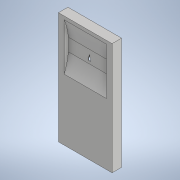
# Autodesk Inventor part: Mosquito Holder v12 RU - Delrin
Saved by Autodesk Inventor 2020 (Build 240168000, 168)
## iProperties
Created: 2016-03-25
Part Number: Mosquito Holder v12 RU - Delrin
Material: Generic
Document SubType Name: Modeling
Designer: Jim
Density: 1 g/cm^3
Appearance: Default
Author: Jim
Autodesk Inventor part; units mm, degrees
ref_plane "XZ Plane" through (0, 0, 0) normal (0, 1, 0) x (-1, 0, 0)
ref_plane "XY Plane" through (0, 0, 0) normal (0, 0, 1) x (1, 0, 0)
sketch "Sketch1" plane through (0, 0, 0) normal (0, 0, 1) x (1, 0, 0)
  line L0 (-3, -3) -> (3, -3)
  line L1 (3, -3) -> (3, 3)
  line L2 (3, 3) -> (-3, 3)
  line L3 (-3, 3) -> (-3, -3)
  line L4 (-3, -3) -> (3, 3) construction
  line L5 (3, -3) -> (-3, 3) construction
  point P0 (0, 0)
  dimension "platform_w" = 6
  dimension "platform_h" = 6
  constraints: 12 end point, 2 midpoint, 2 parallel, 1 horizontal, 1 perpendicular
  measures "platform_w" distance of L2.end L1.end
  measures "platform_h" distance of L1.end L0.end
extrude "Thin_Platform" add sketch "Sketch1" along normal blind 0.1
sketch "Sketch2" plane through (0, 0, 0) normal (0, 0, -1) x (-1, 0, 0)
  line L0 (-0.475, 0) -> (0.475, 0)
  line L1 (0.475, 0) -> (0.475, -1.71)
  line L2 (0.475, -1.71) -> (-0.475, -1.71)
  line L3 (-0.475, -1.71) -> (-0.475, 0)
  line L4 (-0.1663, 0.75) -> (0.1663, 0.75)
  line L5 (0.1663, 0.75) -> (0.1663, 0)
  line L6 (0.1663, 0) -> (-0.1663, 0)
  line L7 (-0.1663, 0) -> (-0.1663, 0.75)
  line L8 (0, -14) -> (0, 14) construction
  line L9 (-4.2, 0) -> (4.2, 0) construction
  point P0 (0, 0)
  point P1 (0, 0)
  point P2 (0, 0)
  dimension "hole_w" = 0.95
  dimension "hole_l" = 1.71
  dimension "organ_channel_l" = 0.75
  dimension "organ_channel_w" = 0.3325
  constraints: 16 end point, 6 midpoint, 4 parallel, 2 horizontal, 2 perpendicular, 1 coincident
  measures "hole_w" distance of L1.end L2.end
  measures "hole_l" distance between parallel lines of L2 L0
  measures "organ_channel_l" distance of L4.end L5.end
  measures "organ_channel_w" distance between parallel lines of L5 L7
extrude "Hole" cut sketch "Sketch2" against normal blind 0.1
sketch "Sketch6" plane through (0, 0, 0.1) normal (0, 0, 1) x (1, 0, 0)
  line L0 (0.1663, 0) -> (0.475, 0) projected
  line L1 (0.475, 0) -> (0.2375, 0)
  line L2 (0.2375, 0) -> (0.2375, -0.3325)
  line L3 (0.2375, -0.3325) -> (0.475, -0.3325)
  line L4 (0.475, -0.3325) -> (0.475, 0)
  point P0 (0, 0)
  dimension "d18" = 0.2375
  dimension "d19" = 0.3325
  constraints: 8 end point, 2 parallel, 1 horizontal, 1 perpendicular
  measures "d18" distance of L3.end L2.end
  measures "d19" distance of L2.end L1.end
extrude "Headrest" add sketch "Sketch6" against normal blind 0.15
mirror "Headrest_mirror" about plane through (0, 0, 0) normal (1, 0, 0) of "Headrest"
sketch "Sketch8" plane through (0, 0, 0) normal (0, 0, -1) x (-1, 0, 0)
  line L0 (0.2375, 0) -> (0.475, 0) projected
  line L1 (0.1663, 0.75) -> (0.1663, 0) projected
  line L2 (0.475, 0) -> (0.1663, 0)
  line L3 (0.1663, 0) -> (0.1663, 0.75)
  line L4 (0.1663, 0.75) -> (0.475, 0.75)
  line L5 (0.475, 0.75) -> (0.475, 0)
  line L6 (-0.2375, 0) -> (-0.475, 0) projected
  line L7 (-0.1663, 0) -> (-0.1663, 0.75) projected
  line L8 (-0.475, 0) -> (-0.1662, 0)
  line L9 (-0.1662, 0) -> (-0.1663, 0.75)
  line L10 (-0.1663, 0.75) -> (-0.475, 0.75)
  line L11 (-0.475, 0.75) -> (-0.475, 0)
  point P0 (0, 0)
  constraints: 16 end point, 4 parallel, 2 horizontal, 2 perpendicular
extrude "Tape_1" add sketch "Sketch8" along normal blind 0.05 draft 0.05
sketch "Sketch9" plane through (0, 0, -0.05) normal (0, 0, -1) x (-1, 0, 0)
  line L0 (-0.475, 0) -> (-0.475, 0.75) projected
  line L1 (0.475, 0) -> (0.475, -0.3325) projected
  line L2 (-0.475, 0.75) -> (0.475, 0.75)
  line L3 (0.475, 0.75) -> (0.475, 0)
  line L4 (0.475, 0) -> (-0.475, 0)
  line L5 (-0.475, 0) -> (-0.475, 0.75)
  point P0 (0, 0)
  constraints: 8 end point, 2 parallel, 1 horizontal, 1 perpendicular
extrude "Wax_Platform" add sketch "Sketch9" along normal blind 0.135
sketch "Sketch27" plane through (0, 0, 0) normal (0, 0, -1) x (-1, 0, 0)
  line L0 (3, 3) -> (-3, 3)
  line L1 (3, -0.3325) -> (3, 3)
  line L2 (-3, 3) -> (-3, -0.3325)
  line L3 (-3, 3) -> (3, 3)
  line L4 (0.475, -0.3325) -> (3, -0.3325)
  line L5 (-3, 3) -> (3, 3) projected
  line L6 (-0.475, -0.3325) -> (-3, -0.3325)
  line L7 (-3, -3) -> (-3, 3) projected
  line L8 (3, 3) -> (3, -3) projected
  line L9 (0.475, 0.75) -> (0.475, 0) projected
  line L10 (0.475, -0.3325) -> (0.475, 0.75)
  line L11 (0.475, 0.75) -> (-0.475, 0.75)
  line L12 (-0.475, 0.75) -> (-0.475, -0.3325)
  point P0 (-0.475, 0.75)
  constraints: 19 end point, 4 perpendicular, 2 collinear, 2 parallel, 1 point on line
extrude "Pillow_Extension" [suppressed]
sketch "Sketch10" plane through (0, 0, 0.1) normal (0, 0, 1) x (1, 0, 0)
  line L0 (3, 3) -> (-3, 3) projected
  line L1 (3, -3) -> (3, 3) projected
  line L2 (-3, 3) -> (-3, -3) projected
  line L3 (-3, -3) -> (3, -3) projected
  line L4 (-10, -10) -> (10, -10)
  line L5 (10, -10) -> (10, 10)
  line L6 (10, 10) -> (-10, 10)
  line L7 (-10, 10) -> (-10, -10)
  line L8 (-10, -10) -> (10, 10) construction
  line L9 (10, -10) -> (-10, 10) construction
  point P0 (0, 0)
  dimension "d27" = 20
  dimension "d28" = 20
  constraints: 12 end point, 2 collinear, 2 midpoint, 1 perpendicular, 1 vertical
  measures "d27" distance of L6.end L5.end
  measures "d28" distance of L5.end L4.end
extrude "Field" add sketch "Sketch10" along normal mid plane 0.5
sketch "Plate_geometry" plane through (0, 0, 0.1) normal (0, 0, 1) x (1, 0, 0)
  line L0 (-12.7, 12.7) -> (12.7, 12.7)
  line L1 (12.7, 12.7) -> (12.7, -40.3)
  line L2 (12.7, -40.3) -> (-12.7, -40.3)
  line L3 (-12.7, -40.3) -> (-12.7, 12.7)
  line L4 (-12.7, 12.7) -> (12.7, -40.3) construction
  line L5 (12.7, 12.7) -> (-12.7, -40.3) construction
  line L6 (0, 23.3) -> (0, -50.9) projected
  line L7 (-114.4038, 0) -> (50.3472, 0) projected
  line L8 (-90.868, 12.7) -> (26.8113, 12.7) construction
  line L9 (-10, -10) -> (10, -10) projected
  line L10 (-10, 10) -> (-10, -10) projected
  line L11 (10, 10) -> (-10, 10) projected
  line L12 (10, -10) -> (10, 10) projected
  point P0 (0, 0)
  point P1 (0, -13.8)
  point P2 (0, -13.8)
  dimension "d31" = 25.4
  dimension "d32" = 53
  dimension "d33" = 12.7
  constraints: 14 end point, 4 midpoint, 3 parallel, 1 collinear, 1 horizontal, 1 perpendicular
  measures "d31" distance of L1.end L2.end
  measures "d32" distance of L0.end L1.end
  measures "d33" distance between parallel lines of L7 L8
extrude "Plate_Extr" add sketch "Plate_geometry" along normal blind 2 and the other way blind 2.5 contours L0 L6 L11 L10 L7 L3 | L0 L1 L7 L12 L11 L6 | L7 L10 L9 L6 L2 L3 | L1 L2 L6 L9 L12 L7
sketch "Organ_Channel" plane through (0, 0, 0.1) normal (0, 0, 1) x (1, 0, 0)
  line L0 (-3, -3) -> (3, -3) projected
  line L1 (3, -3) -> (3, 3) projected
  line L2 (3, 3) -> (-3, 3) projected
  line L3 (-3, 3) -> (-3, -3) projected
  line L4 (0.1662, 0.75) -> (-0.1662, 0.75) projected
  line L5 (0.1663, -0.75) -> (-0.1662, -0.75)
  line L6 (-0.1662, -0.75) -> (-0.1662, 0.75)
  line L7 (-0.1662, 0.75) -> (0.1663, 0.75)
  line L8 (0.1663, 0.75) -> (0.1663, -0.75)
  line L9 (0.1663, -0.75) -> (-0.1662, 0.75) construction
  line L10 (-0.1662, -0.75) -> (0.1663, 0.75) construction
  point P0 (0, 0)
  dimension "d43" = 0.3325
  dimension "d44" = 1.5
  constraints: 12 end point, 2 midpoint, 2 parallel, 1 horizontal, 1 perpendicular
  measures "d43" distance between parallel lines of L6 L8
  measures "d44" distance between parallel lines of L4 L5
sketch "Headrest_Hole" plane through (0, 0, 0.1) normal (0, 0, 1) x (1, 0, 0)
  line L0 (-0.1662, 0) -> (0.1662, 0) projected
  line L1 (-0.2375, 0) -> (-0.1663, 0) projected
  line L2 (-0.2375, 0) -> (-0.2375, -0.3325) projected
  line L3 (-0.2375, -0.3325) -> (-0.475, -0.3325) projected
  line L4 (-0.475, -1.71) -> (-0.475, -0.3325) projected
  line L5 (0.475, -1.71) -> (-0.475, -1.71) projected
  line L6 (0.475, -0.3325) -> (0.475, -1.71) projected
  line L7 (0.2375, -0.3325) -> (0.475, -0.3325) projected
  line L8 (0.2375, 0) -> (0.2375, -0.3325) projected
  line L9 (0.1663, 0) -> (0.2375, 0) projected
  point P0 (0, 0)
sketch "Tape_0" plane through (0, 0, 0) normal (0, 0, -1) x (-1, 0, 0)
  line L0 (3, -3) -> (-3, -3) projected
  line L1 (3, 3) -> (3, -3) projected
  line L2 (-3, -3) -> (-3, 3) projected
  line L3 (0.475, -0.3325) -> (0.475, -1.71) projected
  line L4 (0.475, -1.71) -> (-0.475, -1.71) projected
  line L5 (-0.475, -1.71) -> (-0.475, -0.3325) projected
  line L6 (-0.475, -0.3325) -> (-0.475, 0) projected
  line L7 (-0.475, -0.3325) -> (0.475, -0.3325)
  line L8 (0.475, -0.3325) -> (0.475, 0.75)
  line L9 (0.475, 0.75) -> (-0.475, 0.75)
  line L10 (-0.475, 0.75) -> (-0.475, -0.3325)
  line L11 (-0.475, -0.3325) -> (0.475, 0.75) construction
  line L12 (0.475, -0.3325) -> (-0.475, 0.75) construction
  line L13 (-1.4815, 1.2193) -> (-1.4815, 2.3021)
  line L14 (-1.4815, 2.3021) -> (-2.3274, 2.3021)
  line L15 (-2.3274, 2.3021) -> (-2.3274, 1.2193)
  line L16 (-2.3274, 1.2193) -> (-1.4815, 1.2193)
  line L17 (-1.4815, 1.2193) -> (-2.3274, 2.3021) construction
  line L18 (-1.4815, 2.3021) -> (-2.3274, 1.2193) construction
  line L19 (0, 0.2087) -> (0, 0.75) construction
  line L20 (0.475, 0.75) -> (-0.475, 0.75) construction
  line L21 (0, -14) -> (0, 14) construction
  line L22 (0.1663, 0.75) -> (-0.1663, 0.75) construction
  line L23 (-0.475, -0.3325) -> (-0.2375, -0.3325) construction
  line L24 (-0.475, 0.75) -> (-0.475, 0) construction
  line L25 (0.1663, 0.75) -> (0.475, 0.75) projected
  line L26 (-0.475, 0) -> (-0.475, 0.75) projected
  line L27 (-0.475, 0.75) -> (-0.1663, 0.75) projected
  line L28 (-0.1663, 0.75) -> (0.1663, 0.75) projected
  line L29 (-3, 3) -> (3, 3) projected
  line L30 (0.475, 0.75) -> (0.475, 0) projected
  line L31 (0.475, 0) -> (0.475, -0.3325) projected
  point P0 (-1.9045, 1.7607)
  constraints: 26 end point, 4 midpoint, 4 parallel, 3 collinear, 2 perpendicular, 1 horizontal, 1 point on line, 1 vertical
sketch "Organ_Tape_Face" plane through (0, 0, -0.185) normal (0, 0, -1) x (-1, 0, 0)
  line L0 (0.475, 0.75) -> (-0.475, 0.75) projected
  line L1 (-0.475, 0.75) -> (-0.475, 0) projected
  line L2 (-0.475, 0) -> (0.475, 0) projected
  line L3 (-0.975, 1.25) -> (1, 1.25)
  line L4 (1, 1.25) -> (1, -0.5)
  line L5 (1, -0.5) -> (-0.975, -0.5)
  line L6 (-0.975, -0.5) -> (-0.975, 1.25)
  line L7 (0.475, 0) -> (0.475, 0.75) projected
  point P0 (0, 0)
  dimension "d45" = 0.5
  constraints: 8 end point, 1 other
  measures "d45" distance between parallel lines of L0 L3
sketch "Headrest_Pillows" plane through (0, 0, -0.05) normal (0, 0, -1) x (-1, 0, 0)
  line L0 (0.975, -0.3325) -> (0.975, -1.71)
  line L1 (0.975, -1.71) -> (-1.025, -1.71)
  line L2 (-1.025, -1.71) -> (-1.025, -0.3325)
  line L3 (0.475, -1.71) -> (-0.475, -1.71) projected
  line L4 (-0.475, 0) -> (-0.475, -0.3325) projected
  line L5 (-0.475, -0.3325) -> (-0.2375, -0.3325) projected
  line L6 (-0.2375, -0.3325) -> (-0.2375, 0) projected
  line L7 (0.2375, -0.3325) -> (0.2375, 0) projected
  line L8 (0.475, -0.3325) -> (0.2375, -0.3325) projected
  line L9 (0.475, 0) -> (0.475, -0.3325) projected
  line L10 (-1.025, -0.3325) -> (-0.475, -0.3325)
  line L11 (-0.2375, 0) -> (0.2375, 0)
  line L12 (0.475, -0.3325) -> (0.975, -0.3325)
  line L13 (-0.2375, -0.3325) -> (-0.475, -0.3325) projected
  constraints: 12 end point, 5 point on line, 4 parallel, 3 collinear, 3 perpendicular
sketch "Sketch20" plane through (0, 0, 0) normal (1, 0, 0) x (0, 1, 0)
  line L0 (10, 0.35) -> (10, 2.1)
  line L1 (-10, 0.35) -> (-10, 2.1)
  line L2 (-3, 0) -> (3, 0)
  line L3 (-10, 2.1) -> (10, 2.1)
  ellipse E0 centre (0, 2.1) end of major axis (-10, 2.1) minor radius 2
  line L4 (-10, 0.35) -> (10, 0.35)
  point P0 (0, 0)
  point P1 (0, 0)
  point P2 (0, 0.1)
  constraints: 10 end point, 1 horizontal, 1 midpoint, 4 other
sketch "Sketch21" plane through (0, 0, 0) normal (1, 0, 0) x (0, 1, 0)
  line L0 (0, -6.2139) -> (0, 35.9769) construction
  line L1 (0, 35.9769) -> (0, -6.2139) construction
  line L2 (10, 0.35) -> (10, 2.1) construction
  line L3 (-10, 0.35) -> (10, 0.35) construction
  line L4 (3, 0.35) -> (3, 0.1) projected
  line L5 (-3, 0.1) -> (3, 0.1) projected
  line L6 (-40.3, 2.1) -> (12.7, 2.1) projected
  arc A0 (3, 0.1) -> (11.1534, 2.1) centre (0, 29.9496) ccw
  arc A1 (-11.1534, 2.1) -> (-3, 0.1) centre (0, 29.9496) ccw
  point P0 (0, 0)
  constraints: 4 point on circle, 3 point on line, 2 centre point, 1 end point
sketch "Sketch22" plane through (0, 0, 0) normal (1, 0, 0) x (0, 1, 0)
  line L0 (0, -22.9178) -> (0, 61.0822) construction
  line L1 (0, 61.0822) -> (0, -22.9178) construction
  line L2 (10, 0.35) -> (10, 2.1) construction
  line L3 (-10, 0.35) -> (10, 0.35) construction
  line L4 (3, 0.35) -> (3, 0.1)
  line L5 (-3, 0.1) -> (3, 0.1)
  line L6 (-40.3, 2.1) -> (12.7, 2.1)
  arc A0 (4.8849, 0.35) -> (10, 1.6654) centre (0, 29.9496) ccw
  arc A1 (-10, 1.6654) -> (-4.8849, 0.35) centre (0, 29.9496) ccw
  line L7 (-10, 0.35) -> (10, 0.35) projected
  line L8 (10, 1.6654) -> (10, 0.35)
  line L9 (10, 0.35) -> (4.8849, 0.35)
  line L10 (-10, 0.35) -> (-10, 2.1) projected
  line L11 (-10, 1.6654) -> (-10, 0.35)
  line L12 (-10, 0.35) -> (-4.8849, 0.35)
  point P0 (0, 0)
  point P1 (0, 0)
  constraints: 23 end point, 4 point on circle, 4 point on line, 2 centre point, 1 collinear, 1 perpendicular
extrude "Extrusion10" cut sketch "Sketch21" along normal mid plane 20
extrude "Extrusion11" add sketch "Sketch22" along normal mid plane 20
sketch "Sketch24" plane through (0, 0, -2.4) normal (0, 0, -1) x (-1, 0, 0)
  line L0 (-3, -3) -> (-3, 3) projected
  line L1 (3, 3) -> (3, -3) projected
  line L2 (3, -3) -> (-3, -3) projected
  line L3 (-10, -10) -> (10, -10) projected
  line L4 (10, -10) -> (10, 10) projected
  line L5 (10, 10) -> (-10, 10) projected
  line L6 (-10, 10) -> (-10, -10) projected
  line L7 (12.7, 12.7) -> (12.7, -12.7)
  line L8 (12.7, -12.7) -> (-12.7, -12.7)
  line L9 (-12.7, -12.7) -> (-12.7, 12.7)
  line L10 (-12.7, 12.7) -> (12.7, 12.7)
  line L11 (-3, 3) -> (3, 3) projected
  point P0 (0, 0)
  constraints: 8 end point, 3 other
extrude "Extrusion12" [suppressed]
sketch "Sketch26" plane through (0, 0, -0.05) normal (0, 0, -1) x (-1, 0, 0)
  line L0 (-0.1662, 0.75) -> (-0.1662, 0.75) projected
  line L1 (-0.475, 0) -> (-0.475, 0.75) projected
  line L2 (-0.475, 0) -> (-0.475, 0) projected
  line L3 (-0.475, 0) -> (-0.475, -0.3325) projected
  line L4 (-0.475, -0.3325) -> (-0.2375, -0.3325) projected
  line L5 (-0.2375, -0.3325) -> (-0.2375, 0) projected
  line L6 (-0.1662, 0) -> (-0.2375, 0) projected
  line L7 (0.1662, 0) -> (0.1662, 0) projected
  line L8 (0.2375, 0) -> (0.1662, 0) projected
  line L9 (0.2375, -0.3325) -> (0.2375, 0) projected
  line L10 (0.475, -0.3325) -> (0.2375, -0.3325) projected
  line L11 (-0.475, 0) -> (-0.475, -0.3325) projected
  line L12 (-0.2375, -0.3325) -> (-0.475, -0.3325)
  line L13 (-0.475, -0.3325) -> (-0.475, 0)
  line L14 (-0.475, 0) -> (-0.2375, 0)
  line L15 (-0.2375, 0) -> (-0.2375, -0.3325)
  line L16 (0.475, -0.3325) -> (0.2375, -0.3325) projected
  line L17 (0.2375, -0.3325) -> (0.2375, 0) projected
  line L18 (0.475, -0.3325) -> (0.2375, -0.3325)
  line L19 (0.2375, -0.3325) -> (0.2375, 0)
  line L20 (0.2375, 0) -> (0.475, 0)
  line L21 (0.475, 0) -> (0.475, -0.3325)
  line L22 (0.475, 0) -> (0.1662, 0) projected
  line L23 (0.475, 0) -> (0.1662, 0) projected
  line L24 (0.1662, 0.75) -> (0.475, 0.75) projected
  line L25 (0.1662, 0.75) -> (0.1662, 0.75) projected
  line L26 (0.1662, 0.75) -> (0.475, 0.75) projected
  line L27 (-0.475, 0.75) -> (-0.1662, 0.75) projected
  line L28 (-0.1662, 0.75) -> (-0.1662, 0.75) projected
  line L29 (-0.475, 0.75) -> (-0.1662, 0.75) projected
  line L30 (-0.475, 0) -> (-0.475, 0.75) projected
  line L31 (-0.475, 0) -> (-0.475, 0) projected
  line L32 (-0.475, 0) -> (-0.475, -0.3325) projected
  line L33 (-0.475, -0.3325) -> (-0.2375, -0.3325) projected
  line L34 (-0.2375, -0.3325) -> (-0.2375, 0) projected
  line L35 (-0.1662, 0) -> (-0.2375, 0) projected
  line L36 (-0.1662, 0) -> (-0.1662, 0) projected
  line L37 (-0.475, 0) -> (-0.475, 0.75) projected
  line L38 (-0.475, 0.75) -> (-0.1662, 0.75) projected
  line L39 (-0.475, 0.75) -> (-0.1662, 0.75) projected
  line L40 (-0.1662, 0) -> (-0.1662, 0) projected
  line L41 (-0.475, 0) -> (-0.475, 0.75) projected
  line L42 (0.1662, 0) -> (0.1662, 0) projected
  line L43 (0.2375, 0) -> (0.1662, 0) projected
  line L44 (0.2375, -0.3325) -> (0.2375, 0) projected
  line L45 (0.475, -0.3325) -> (0.2375, -0.3325) projected
  line L46 (0.1662, 0.75) -> (0.475, 0.75) projected
  line L47 (0.1662, 0.75) -> (0.1662, 0.75) projected
  line L48 (0.1662, 0.75) -> (0.475, 0.75) projected
  line L49 (-0.2375, -0.3325) -> (-0.475, -0.3325)
  line L50 (-0.475, -0.3325) -> (-0.475, 0)
  line L51 (-0.475, 0) -> (-0.2375, 0)
  line L52 (-0.2375, 0) -> (-0.2375, -0.3325)
  line L53 (0.2375, -0.3325) -> (0.475, -0.3325)
  line L54 (0.475, -0.3325) -> (0.475, 0)
  line L55 (0.475, 0) -> (0.2375, 0)
  line L56 (0.2375, 0) -> (0.2375, -0.3325)
  line L57 (-0.1662, 0) -> (-0.475, 0) projected
  line L58 (0.475, 0) -> (0.475, -0.3325) projected
  line L59 (0.475, 0) -> (0.475, 0) projected
  line L60 (0.475, 0.75) -> (0.475, 0) projected
  line L61 (0.475, 0.75) -> (0.475, 0) projected
  line L62 (-0.1662, 0) -> (-0.475, 0) projected
  line L63 (0.475, 0) -> (0.475, -0.3325) projected
  line L64 (0.475, 0) -> (0.475, 0) projected
  line L65 (0.475, 0.75) -> (0.475, 0) projected
  line L66 (0.475, 0.75) -> (0.475, 0) projected
  point P0 (0, 0)
  constraints: 32 end point, 8 parallel, 4 horizontal, 4 perpendicular
extrude "Extrusion13" [suppressed]
sketch "Sketch28" plane through (-0.1662, 0, -0.05) normal (0, 0, -1) x (-1, 0, 0)
  line L0 (0.0713, 0) -> (0.0713, -0.3325) projected
  line L1 (0.3087, -0.3325) -> (0.3087, 0) projected
  line L2 (0.0713, -0.3325) -> (0.3087, -0.3325)
  line L3 (0.3087, -0.3325) -> (0.3087, 0)
  line L4 (0.3087, 0) -> (0.0713, 0)
  line L5 (0.0713, 0) -> (0.0713, -0.3325)
  line L6 (-0.6412, 0) -> (-0.6412, 0.75) projected
  line L7 (-0.4037, -0.3325) -> (-0.6412, -0.3325)
  line L8 (-0.6412, -0.3325) -> (-0.6412, 0)
  line L9 (-0.6412, 0) -> (-0.4037, 0)
  line L10 (-0.4037, 0) -> (-0.4037, -0.3325)
  line L11 (-0.4037, -0.3325) -> (-0.4037, 0) projected
  point P0 (-0.1662, 0)
  constraints: 16 end point, 4 parallel, 2 horizontal, 2 perpendicular, 1 collinear, 1 point on line
extrude "Extrusion15" add sketch "Sketch28" along normal up to surface (0.135 mm away)
sketch "Sketch29" plane through (0, 0, 0) normal (0, 0, -1) x (-1, 0, 0)
  line L0 (-3, -3) -> (-3, 3) projected
  line L1 (3, 3) -> (3, -3) projected
  line L2 (-3, 3) -> (3, 3)
  line L3 (3, 3) -> (3, -0.3325)
  line L4 (-3, -0.3325) -> (-3, 3)
  line L5 (-0.2375, -0.3325) -> (-0.475, -0.3325) projected
  line L6 (-0.475, 0.75) -> (-0.475, -0.3325) projected
  line L7 (0.475, 0) -> (0.475, -0.3325) projected
  line L8 (-0.475, 0.75) -> (0.475, 0.75)
  line L9 (0.475, 0.75) -> (0.475, -0.3325)
  line L10 (-0.475, -0.3325) -> (-0.475, 0.75)
  line L11 (3, -0.3325) -> (0.475, -0.3325)
  line L12 (-0.475, -0.3325) -> (-3, -0.3325)
  point P0 (0, 0)
  constraints: 16 end point, 4 parallel, 2 collinear, 2 horizontal, 2 perpendicular, 1 point on line
extrude "Extrusion16" add sketch "Sketch29" along normal up to surface (0.185 mm away)
ref_plane "Work Plane1" through (0, 0, -6.2956) normal (0, 0, -1) x (-1, 0, 0)
ref_plane "Work Plane2" through (-12.7, -13.8, 2.1) normal (0, 1, 0) x (1, 0, 0)
sketch "Sketch30" plane through (0, 0, -2.4) normal (0, 0, -1) x (-1, 0, 0)
  line L0 (7.75, -10) -> (7.75, -40.3) construction
  line L1 (-12.7, -40.3) -> (12.7, -40.3) construction
  line L2 (10, -10) -> (-10, -10) construction
  line L3 (0, -25.15) -> (36.8265, -25.15) construction
  line L4 (0, -10) -> (0, -40.3) construction
  line L5 (9.3851, -15.3393) -> (9.3851, -34.9608) construction
  line L6 (7.75, -15.3393) -> (7.75, -34.9608)
  line L7 (11.0202, -34.9608) -> (11.0202, -15.3393)
  arc A0 (11.0202, -15.3393) -> (7.75, -15.3393) centre (9.3851, -15.3393) ccw
  arc A1 (7.75, -34.9608) -> (11.0202, -34.9608) centre (9.3851, -34.9608) ccw
  point P0 (0, 0)
  point P1 (9.3851, -25.15)
  dimension "d70" = 7.75
  dimension "d73" = 3.2702
  dimension "d74" = 19.6215
  constraints: 14 end point, 4 midpoint, 4 point on circle, 4 tangent, 3 point on line, 3 vertical, 2 centre point, 1 collinear, 1 horizontal, 1 parallel
  measures "d70" distance between parallel lines of L4 L0
  measures "d73" diameter of A1
  measures "d74" distance of L5.end L5.start
extrude "Extrusion17" cut sketch "Sketch30" against normal blind 4.064
mirror "Mirror3" about plane through (0, 0, 0) normal (1, 0, 0) of "Extrusion17"
equation "\"organ_channel_w\" = 0.35 * hole_w"
equation "\"d18\" = 0.25 * hole_w"
equation "\"d19\" = 1.4 * d18"
equation "\"head_rest\" = 1.5 * platform_th"
equation "\"d23\" = head_rest - platform_th"
equation "\"d43\" = organ_channel_w"
equation "\"d44\" = 2 * organ_channel_l"
equation "\"platform_th\" = 0.1"
body "Solid1"
